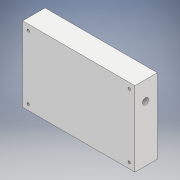
# Autodesk Inventor part: USB-1SP16T-83H-01
Saved by Autodesk Inventor 2018 (Build 220112000, 112)
## iProperties
Created: 2019-09-24
Part Number: USB-1SP16T-83H-01
Material: Generic
Document SubType Name: Modeling
Designer: alexanderpollak
Density: 1 g/cm^3
Appearance: Denim - Blue
Author: alexanderpollak
Autodesk Inventor part; units mm, degrees
ref_plane "YZ Plane" through (0, 0, 0) normal (1, 0, 0) x (0, 1, 0)
ref_plane "XZ Plane" through (0, 0, 0) normal (0, 1, 0) x (-1, 0, 0)
ref_plane "XY Plane" through (0, 0, 0) normal (0, 0, 1) x (1, 0, 0)
sketch "Sketch1" plane through (0, 0, 0) normal (0, 1, 0) x (-1, 0, 0)
  line L0 (38.1, 25.4) -> (-38.1, 25.4)
  line L1 (-38.1, 25.4) -> (-38.1, -25.4)
  line L2 (-38.1, -25.4) -> (38.1, -25.4)
  line L3 (38.1, -25.4) -> (38.1, 25.4)
  line L4 (38.1, 25.4) -> (-38.1, -25.4) construction
  line L5 (-38.1, 25.4) -> (38.1, -25.4) construction
  point P0 (0, 0)
  dimension "d0" = 76.2
  dimension "d1" = 50.8
  constraints: 12 end point, 2 midpoint, 2 parallel, 1 horizontal, 1 perpendicular
  measures "d0" distance of L2.end L1.end
  measures "d1" distance between parallel lines of L0 L2
extrude "Extrusion1" add sketch "Sketch1" along normal blind 15.2
sketch "Sketch5" plane through (0, 0, 0) normal (0, -1, 0) x (1, 0, 0)
  line L0 (-34.29, -21.59) -> (34.29, -21.59) construction
  line L1 (34.29, -21.59) -> (34.29, 21.59) construction
  line L2 (34.29, 21.59) -> (-34.29, 21.59) construction
  line L3 (-34.29, 21.59) -> (-34.29, -21.59) construction
  line L4 (-34.29, -21.59) -> (34.29, 21.59) construction
  line L5 (34.29, -21.59) -> (-34.29, 21.59) construction
  point P0 (0, 0)
  dimension "d44" = 68.58
  dimension "d45" = 43.18
  constraints: 12 end point, 4 coincident, 2 midpoint, 2 parallel, 1 horizontal, 1 perpendicular
  measures "d44" distance of L2.end L1.end
  measures "d45" distance of L1.end L0.end
hole "Hole5" at (-34.29, 0, 21.59) at (34.29, 0, 21.59) at (34.29, 0, -21.59) at (-34.29, 0, -21.59) direction (0, 1, 0) diameter 1.694 depth 6.35 tip angle 118 thread size "2-56 UNC" class "2B" standard "ANSI Unified Screw Threads"
sketch "Sketch6" plane through (38.1, 0, 25.4) normal (1, 0, 0) x (0, 0, -1)
  line L0 (0, 0) -> (50.8, 0) projected
  line L1 (0, 0) -> (0, 15.2) projected
  point P0 (25.4, 0)
  point P1 (12.7, 7.1)
  dimension "d60" = 7.1
  dimension "d61" = 12.7
  measures "d60" distance from line of point (12.7, 7.1) L0
  measures "d61" distance from line of point (12.7, 7.1) L1
hole "Hole6" at (38.1, 7.1, 12.7) direction (-1, 0, 0) diameter 4.077 depth 5
sketch "Sketch7" plane through (-38.1, 0, -25.4) normal (-1, 0, 0) x (0, 0, 1)
  circle A0 centre (38.1, 7.1) radius 2.0385 projected
  point P0 (25.4, 0)
  constraints: 1 coincident
hole "Hole7" at (-38.1, 7.1, 12.7) direction (1, 0, 0) diameter 4.077 depth 5
body "Solid1"
